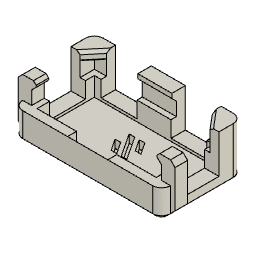
Heatbed Terminal Cover (Autodesk Fusion 360 design; units mm, degrees)
Autodesk Fusion 360 part; units mm, degrees
sketch "Sketch1" plane through (0, 0, 0) normal (0, 0, 1) x (1, 0, 0)
  line L0 (16.5, 8) -> (-16.5, 8)
  line L1 (-16.5, 8) -> (-16.5, -8)
  line L2 (-16.5, -8) -> (16.5, -8)
  line L3 (16.5, -8) -> (16.5, 8)
  line L4 (16.5, 8) -> (-16.5, -8) construction
  line L5 (-16.5, 8) -> (16.5, -8) construction
  line L6 (0, -2) -> (0, 0) construction
  dimension "d2" = 33
  dimension "d3" = 16
  dimension "d28" = 2
  constraint horizontal L0
  constraint perpendicular L0 L1
  constraint parallel L0 L2
  constraint parallel L1 L3
  constraint coincident L4 L6.end
  constraint coincident L5 L6.end
  constraint coincident L6.end origin
  constraint vertical L6
  measures "d2" distance of L0.start L0.end
  measures "d3" distance of L0.start L2.end
  measures "d28" distance of L6.start L6.end
extrude "Extrude1" add sketch "Sketch1" along normal blind 2
sketch "Sketch2" plane through (0, 0, 2) normal (0, 0, 1) x (-1, 0, 0)
  line L0 (-16.5, 8) -> (-16.5, -8)
  line L1 (-16.5, -8) -> (16.5, -8)
  line L2 (16.5, -8) -> (16.5, 8)
  line L3 (16.5, 8) -> (-16.5, 8)
  line L4 (13.3, 8) -> (13.3, -4.8)
  line L5 (13.3, -4.8) -> (-13.3, -4.8)
  line L6 (-13.3, -4.8) -> (-13.3, 8)
  dimension "d6" = 3.2
  dimension "d7" = 3.2
  dimension "d8" = 3.2
  constraint coincident L3 L4.start
  constraint perpendicular L3 L4
  constraint perpendicular L4 L5
  constraint coincident L3 L6.end
  constraint perpendicular L3 L6
  measures "d6" distance of L0 L6
  measures "d7" distance of L2 L4
  measures "d8" distance of L1 L5
extrude "Extrude2" add sketch "Sketch2" along normal blind 4.2 contours L0 L1 L2 L3 L4 L5 L6
sketch "Sketch3" plane through (0, 0, 6.2) normal (0, 0, 1) x (-1, 0, 0)
  line L0 (-13.3, -4.8) -> (-13.3, 8)
  line L1 (-13.3, 8) -> (-16.5, 8)
  line L2 (-16.5, 8) -> (-16.5, -8)
  line L3 (-16.5, -8) -> (16.5, -8)
  line L4 (16.5, -8) -> (16.5, 8)
  line L5 (16.5, 8) -> (13.3, 8)
  line L6 (13.3, 8) -> (13.3, -4.8)
  line L7 (13.3, -4.8) -> (-13.3, -4.8)
  line L8 (14.5, 8) -> (14.5, -6)
  line L9 (14.5, -6) -> (-14.5, -6)
  line L10 (-14.5, -6) -> (-14.5, 8)
  dimension "d11" = 2
  dimension "d12" = 2
  dimension "d13" = 2
  constraint coincident L5 L8.start
  constraint perpendicular L5 L8
  constraint perpendicular L8 L9
  constraint coincident L1 L10.end
  constraint perpendicular L1 L10
  measures "d11" distance of L2 L10
  measures "d12" distance of L3 L9
  measures "d13" distance of L4 L8
extrude "Extrude3" add sketch "Sketch3" along normal blind 3 contours L1 L2 L3 L4 L5 L8 L9 L10
sketch "Sketch4" plane through (0, 0, 2) normal (0, 0, 1) x (-1, 0, 0)
  line L0 (13.3, -4.8) -> (13.3, 8)
  line L1 (13.3, 8) -> (-13.3, 8)
  line L2 (-13.3, 8) -> (-13.3, -4.8)
  line L3 (-13.3, -4.8) -> (13.3, -4.8)
  line L4 (2.5, 8) -> (-2.5, 8)
  line L5 (-2.5, 8) -> (-2.5, 5)
  line L6 (-2.5, 5) -> (2.5, 5)
  line L7 (2.5, 5) -> (2.5, 8)
  dimension "d16" = 3
  dimension "d17" = 5
  constraint horizontal L4
  constraint vertical L5
  constraint horizontal L6
  constraint vertical L7
  constraint coincident L1 L4.start
  constraint midpoint L1 L4
  measures "d16" distance of L4.end L5.end
  measures "d17" distance of L5.end L6.end
sketch "Sketch5" plane through (0, 0, 2) normal (0, 0, 1) x (-1, 0, 0)
  line L0 (-13.3, 8) -> (-13.3, -4.8)
  line L1 (-13.3, -4.8) -> (13.3, -4.8)
  line L2 (13.3, -4.8) -> (13.3, 8)
  line L3 (13.3, 8) -> (-13.3, 8)
  line L4 (-13.3, -2.8) -> (-18.3, -2.8)
  line L5 (-18.3, -2.8) -> (-18.3, 5.2)
  line L6 (-18.3, 5.2) -> (-13.3, 5.2)
  line L7 (-13.3, 5.2) -> (-13.3, -2.8)
  line L8 (13.3, 5.2) -> (18.3, 5.2)
  line L9 (18.3, 5.2) -> (18.3, -2.8)
  line L10 (18.3, -2.8) -> (13.3, -2.8)
  line L11 (13.3, -2.8) -> (13.3, 5.2)
  line L12 (3.8, -4.8) -> (11.8, -4.8)
  line L13 (11.8, -4.8) -> (11.8, -9.8)
  line L14 (11.8, -9.8) -> (3.8, -9.8)
  line L15 (3.8, -9.8) -> (3.8, -4.8)
  line L16 (-3.8, -4.8) -> (-11.8, -4.8)
  line L17 (-11.8, -4.8) -> (-11.8, -9.8)
  line L18 (-11.8, -9.8) -> (-3.8, -9.8)
  line L19 (-3.8, -9.8) -> (-3.8, -4.8)
  dimension "d20" = 5
  dimension "d21" = 2
  dimension "d22" = 2
  dimension "d23" = 8
  dimension "d24" = 1.5
  dimension "d25" = 1.5
  constraint horizontal L4
  constraint vertical L5
  constraint horizontal L6
  constraint vertical L7
  constraint coincident L0 L4.start
  constraint horizontal L8
  constraint vertical L9
  constraint horizontal L10
  constraint vertical L11
  constraint coincident L2 L8.start
  constraint horizontal L12
  constraint vertical L13
  constraint horizontal L14
  constraint vertical L15
  constraint coincident L1 L12.start
  constraint horizontal L16
  constraint vertical L17
  constraint horizontal L18
  constraint vertical L19
  constraint coincident L1 L16.start
  constraint equal L6 L8
  constraint equal L13 L19
  constraint equal L6 L19
  constraint equal L9 L14
  constraint equal L14 L18
  constraint equal L5 L18
  measures "d20" distance of L5.end L6.end
  measures "d21" distance of L1.end L10.end
  measures "d22" distance of L0.end L4.start
  measures "d23" distance of L4.end L5.end
  measures "d24" distance of L1.end L12.end
  measures "d25" distance of L0.end L16.end
extrude "Extrude5" cut sketch "Sketch5" along normal through all from surface at 0.6 contours L0 L4 L5 L6 L7 | L2 L8 L9 L10 L11 | L1 L16 L17 L18 L19 | L1 L12 L13 L14 L15
sketch "Sketch6" plane through (0, -8, 0) normal (0, -1, 0) x (1, 0, 0)
  line L0 (13.3, 2) -> (-13.3, 2) construction
  line L1 (-13.3, 2) -> (-13.3, 6.2)
  line L2 (-13.3, 6.2) -> (-14.5, 6.2)
  line L3 (-14.5, 6.2) -> (-14.5, 9.2)
  line L4 (-14.5, 9.2) -> (-16.5, 9.2)
  line L5 (-16.5, 9.2) -> (-16.5, 0)
  line L6 (-16.5, 0) -> (16.5, 0)
  line L7 (16.5, 0) -> (16.5, 9.2)
  line L8 (16.5, 9.2) -> (14.5, 9.2)
  line L9 (14.5, 9.2) -> (14.5, 6.2)
  line L10 (14.5, 6.2) -> (13.3, 6.2)
  line L11 (13.3, 6.2) -> (13.3, 2)
  line L12 (-16.5, 6.2) -> (16.5, 6.2)
  line L13 (16.5, 6.2) -> (16.5, 0)
  line L14 (16.5, 0) -> (-16.5, 0)
  line L15 (-16.5, 0) -> (-16.5, 6.2)
  line L16 (13.3, 0) -> (13.3, 1.1)
  line L17 (13.3, 1.1) -> (13.3, 6.2)
  line L18 (2.5, 6.2) -> (2.5, 0)
  constraint horizontal L12
  constraint vertical L13
  constraint horizontal L14
  constraint vertical L15
  constraint coincident L6.end L7.start
  constraint coincident L5 L12.start
  constraint coincident L10.end L12
  constraint coincident L6 L16.start
  constraint perpendicular L6 L16
  constraint coincident L12 L10.end
  constraint perpendicular L12 L17
  constraint coincident L12 L18.start
  constraint coincident L14 L18.end
  constraint perpendicular L14 L18
  constraint coincident L0.start L17
extrude "Extrude6" add sketch "Sketch6" along normal blind 2 contours L2 L5 L6 L12 L14 L15 L18 | L6 L11 L12 L14 L16 L17 L18 | L6 L7 L10 L11 L12 L13 L14 L16 L17
fillet "Fillet1" radius 2 4 edges at (-16.5, -10, 3.1) (-16.5, 8, 4.6) (16.5, -10, 3.1) (16.5, 8, 4.6)
chamfer "Chamfer1" distance 0.8 angle 45 9 edges at (-16.5, -1, 0) (-15.9142, -9.4142, 0) (0, -10, 0) (0, -10, 0) (15.9142, -9.4142, 0) (16.5, -1, 0) (15.9142, 7.4142, 0) (0, 8, 0) (-15.9142, 7.4142, 0)
sketch "Sketch8" plane through (0, 0, 9.2) normal (0, 0, 1) x (-1, 0, 0)
  arc A0 (14.5, -8) -> (16.5, -6) centre (14.5, -6) ccw
  line L0 (16.5, -6) -> (16.5, -2.8)
  line L1 (16.5, -2.8) -> (14.5, -2.8)
  line L2 (14.5, -2.8) -> (14.5, -6)
  line L3 (14.5, -6) -> (11.8, -6) construction
  line L4 (11.8, -6) -> (11.8, -8)
  line L5 (11.8, -8) -> (14.5, -8)
  line L6 (3.8, -8) -> (3.8, -6)
  line L7 (3.8, -6) -> (-3.8, -6) construction
  line L8 (-3.8, -6) -> (-3.8, -8)
  line L9 (-3.8, -8) -> (3.8, -8)
  arc A1 (-16.5, -6) -> (-14.5, -8) centre (-14.5, -6) ccw
  line L10 (-14.5, -8) -> (-11.8, -8)
  line L11 (-11.8, -8) -> (-11.8, -6)
  line L12 (-11.8, -6) -> (-14.5, -6)
  line L13 (-14.5, -6) -> (-14.5, -2.8) construction
  line L14 (-14.5, -2.8) -> (-16.5, -2.8)
  line L15 (-16.5, -2.8) -> (-16.5, -6)
  line L16 (-16.5, 5.2) -> (-14.5, 5.2)
  line L17 (-14.5, 5.2) -> (-14.5, 8) construction
  line L18 (-14.5, 8) -> (-16.5, 8)
  line L19 (-16.5, 8) -> (-16.5, 5.2)
  line L20 (14.5, 5.2) -> (16.5, 5.2)
  line L21 (16.5, 5.2) -> (16.5, 8)
  line L22 (16.5, 8) -> (14.5, 8)
  line L23 (14.5, 8) -> (14.5, 5.2) construction
  line L24 (16.5, 8) -> (13.5, 8)
  line L25 (13.5, 8) -> (13.5, 5.2)
  line L26 (13.5, 5.2) -> (16.5, 5.2)
  line L27 (16.5, 5.2) -> (16.5, 8)
  line L28 (-16.5, 8) -> (-13.5, 8)
  line L29 (-13.5, 8) -> (-13.5, 5.2)
  line L30 (-13.5, 5.2) -> (-16.5, 5.2)
  line L31 (-16.5, 5.2) -> (-16.5, 8)
  line L32 (3.8, -8) -> (-3.8, -8)
  line L33 (-3.8, -8) -> (-3.8, -5)
  line L34 (-3.8, -5) -> (3.8, -5)
  line L35 (3.8, -5) -> (3.8, -8)
  line L36 (14.5, -2.8) -> (11.8, -6)
  line L37 (-11.8, -6) -> (-14.5, -2.8)
  dimension "d35" = 1
  constraint horizontal L24
  constraint vertical L25
  constraint horizontal L26
  constraint vertical L27
  constraint coincident L21.end L22.start
  constraint horizontal L28
  constraint vertical L29
  constraint horizontal L30
  constraint vertical L31
  constraint coincident L18.end L19.start
  constraint horizontal L32
  constraint vertical L33
  constraint horizontal L34
  constraint vertical L35
  constraint coincident L6.start L9.end
  constraint coincident L7.end L33
  constraint coincident L16.start L30
  constraint coincident L20.end L21.start
  constraint equal L26 L30
  constraint equal L26 L35
  constraint coincident L1.end L2.start
  constraint coincident L3.end L4.start
  constraint coincident L11.end L12.start
  constraint coincident L13.end L14.start
  measures "d35" horizontal distance of L16.end L29.end
extrude "Extrude7" add sketch "Sketch8" along normal blind 2
chamfer "Chamfer2" distance 1 angle 45 3 edges at (0, 5, 9.2) (-13.5, -6.6, 9.2) (13.5, -6.6, 9.2)
chamfer "Chamfer3" distance 0.4 angle 45 2 edges at (13.15, 4.4, 9.2) (-13.15, 4.4, 9.2)
sketch "Sketch9" plane through (0, 0, 0) normal (0, 0, -1) x (1, 0, 0)
  line L0 (14.5, 9.2) -> (-14.5, 9.2)
  arc A0 (-14.5, 9.2) -> (-15.7, 8) centre (-14.5, 8) ccw
  line L1 (-15.7, 8) -> (-15.7, -6)
  arc A1 (-15.7, -6) -> (-14.5, -7.2) centre (-14.5, -6) ccw
  line L2 (-14.5, -7.2) -> (14.5, -7.2)
  arc A2 (14.5, -7.2) -> (15.7, -6) centre (14.5, -6) ccw
  line L3 (15.7, -6) -> (15.7, 8)
  arc A3 (15.7, 8) -> (14.5, 9.2) centre (14.5, 8) ccw
  line L4 (-15.7, 1) -> (15.7, 1) construction
  line L5 (2.327, 3.591) -> (-1.077, -1.591)
  line L6 (-0.625, 1) -> (0.625, 1) construction
  line L7 (-2.327, -1.591) -> (1.077, 3.591)
  line L8 (1.077, 3.591) -> (2.327, 3.591)
  line L9 (-2.327, -1.591) -> (-1.077, -1.591)
  line L10 (-1.077, -1.591) -> (-0.077, -1.591) construction
  line L11 (-0.077, -1.591) -> (1.625, 1)
  line L12 (1.625, 1) -> (2.875, 1)
  line L13 (2.875, 1) -> (1.173, -1.591)
  line L14 (1.173, -1.591) -> (-0.077, -1.591)
  line L15 (-0.625, 1) -> (-1.625, 1) construction
  line L16 (-1.625, 1) -> (0.077, 3.591)
  line L17 (0.077, 3.591) -> (-1.173, 3.591)
  line L18 (-1.173, 3.591) -> (-2.875, 1)
  line L19 (-1.625, 1) -> (-2.875, 1)
  point P0 (0, 1)
  dimension "d40" = 6.2
  dimension "d41" = 1.25
  dimension "d42" = 56.7
  dimension "d43" = 1
  dimension "d44" = 1
  constraint midpoint L1 L4.start
  constraint midpoint L3 L4.end
  constraint midpoint L4 P0
  constraint coincident L4 L6.start
  constraint coincident L4 L6.end
  constraint midpoint P0 L6
  constraint midpoint L5 L6.end
  constraint equal L5 L7
  constraint midpoint L6.start L7
  constraint parallel L5 L7
  constraint parallel L9 L10
  constraint coincident L4 L11.end
  constraint coincident L4 L12.end
  constraint parallel L4 L12
  constraint parallel L11 L13
  constraint parallel L5 L11
  constraint equal L11 L13
  constraint equal L9 L14
  constraint coincident L4 L15.end
  constraint parallel L15 L17
  constraint coincident L4 L18.end
  constraint parallel L16 L18
  constraint parallel L4 L19
  constraint equal L8 L19
  constraint parallel L7 L16
  constraint equal L11 L16
  measures "d40" distance of L5.start L5.end
  measures "d41" distance of L6.start L6.end
  measures "d42" angle of L4 L5
  measures "d43" distance of L5.end L10.end
  measures "d44" distance of L6.start L15.end
extrude "Extrude8" cut sketch "Sketch9" against normal through all from surface at -0.2 contours L5 L7 L8 L9 | L11 L12 L13 L14 | L16 L17 L18 L19
sketch "Sketch11" plane through (0, 0, 0) normal (1, 0, 0) x (0, 1, 0)
  line L0 (-10, 6.2) -> (-8, 6.2)
  line L1 (-8, 6.2) -> (-8, 4.2)
  line L2 (-8, 4.2) -> (-10, 6.2)
  point P0 (-8, 6.2)
  point P1 (-10, 6.2)
  dimension "d48" = 2
  constraint coincident P1 L0.start
  constraint coincident P0 L0.end
  constraint perpendicular L0 L1
  measures "d48" distance of P0 L1.end
extrude "Extrude9" cut sketch "Sketch11" along normal mid plane 9
chamfer "Chamfer4" distance 0.6 angle 45 4 edges at (13.5, -6.6, 11.2) (-13.5, -6.6, 11.2) (13.15, 4.4, 11.2) (-13.15, 4.4, 11.2)
sketch "Sketch12" plane through (0, -5.2, 0) normal (0, 1, 0) x (-1, 0, 0)
  line L0 (14.1, 11.2) -> (13.5, 10.6)
  line L1 (13.5, 10.6) -> (13.5, 10.2)
  line L2 (13.5, 10.2) -> (14.5, 9.2)
  line L3 (14.5, 9.2) -> (14.5, 6.2)
  line L4 (14.5, 6.2) -> (13.3, 6.2)
  line L5 (13.3, 6.2) -> (13.3, 2.6)
  line L6 (13.3, 2.6) -> (16.5, 2.6)
  line L7 (16.5, 2.6) -> (16.5, 11.2)
  line L8 (16.5, 11.2) -> (14.1, 11.2)
  line L9 (16.5, 11.2) -> (17.5, 10.2)
  line L10 (17.5, 10.2) -> (17.5, 1.8)
  line L11 (17.5, 1.8) -> (16.5, 0.8)
  line L12 (16.5, 0.8) -> (16.5, 2.6)
  line L13 (-13.5, 10.6) -> (-14.1, 11.2)
  line L14 (-14.1, 11.2) -> (-16.5, 11.2)
  line L15 (-16.5, 11.2) -> (-16.5, 2.6)
  line L16 (-16.5, 2.6) -> (-13.3, 2.6)
  line L17 (-13.3, 2.6) -> (-13.3, 6.2)
  line L18 (-13.3, 6.2) -> (-14.5, 6.2)
  line L19 (-14.5, 6.2) -> (-14.5, 9.2)
  line L20 (-14.5, 9.2) -> (-13.5, 10.2)
  line L21 (-13.5, 10.2) -> (-13.5, 10.6)
  line L22 (-13.3, 2.6) -> (13.3, 2.6) construction
  line L23 (0, 2.6) -> (0, 19.8821) construction
  line L24 (-17.5, 1.8) -> (-16.5, 0.8)
  line L25 (-16.5, 0.8) -> (-16.5, 2.6)
  line L26 (-16.5, 11.2) -> (-17.5, 10.2)
  line L27 (-17.5, 10.2) -> (-17.5, 1.8)
  point P0 (16.5, 0.8)
  dimension "d52" = 45
  dimension "d54" = 1
  dimension "d55" = 45
  constraint coincident L7.end L8.start
  constraint coincident P0 L11.end
  constraint coincident L6.end L7.start
  constraint parallel L7 L10
  constraint coincident L16.end L17.start
  constraint coincident L5.end L6.start
  constraint midpoint L22 L23.start
  constraint perpendicular L22 L23
  constraint symmetric L7.end L23 L14.end
  constraint symmetric L9.end L23 L26.end
  constraint symmetric L10.end L23 L24.start
  constraint symmetric P0 L23 L24.end
  constraint symmetric L6.end L23 L15.end
  measures "d52" angle of L7 L9
  measures "d54" distance of L7 L10
  measures "d55" angle of L11 L12
extrude "Extrude10" add sketch "Sketch12" against normal up to surface (2.8 mm away) contours L7 L9 L10 L11 L12 | L15 L24 L25 L26 L27
equation "d2 = 29 mm + 4 mm"
equation "d3 = 14 mm + 2 mm"
named bodies: "Cover"
